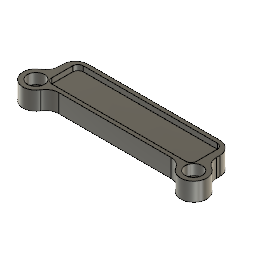
nametag (Autodesk Fusion 360 design; units mm, degrees)
Autodesk Fusion 360 part; units mm, degrees
note: some values were not read from the file. Set by a fixed rule: which sketch regions a step uses.
sketch "Sketch1" plane through (0, 0, 0) normal (0, 0, 1) x (1, 0, 0) in component "node_nametag"
  circle A0 centre (-64.8296, 1.0244) radius 1.75
  circle A1 centre (-4.8296, 1.0244) radius 1.75
  circle A2 centre (-64.8296, 1.0244) radius 5
  circle A3 centre (-4.8296, 1.0244) radius 5
  line L0 (-64.8296, 16.0244) -> (-4.8296, 16.0244)
  line L1 (-4.8296, 16.0244) -> (-4.8296, 1.0244)
  line L2 (-4.8296, 1.0244) -> (-64.8296, 1.0244)
  line L3 (-64.8296, 1.0244) -> (-64.8296, 16.0244)
  dimension "d1" = 3.5
  dimension "d2" = 3.5
  dimension "d3" = 60
  dimension "d4" = 10
  dimension "d5" = 10
  dimension "d6" = 15
  constraint horizontal A0.centre A1.centre
  constraint concentric A0 A2
  constraint concentric A1 A3
  constraint horizontal L0
  constraint vertical L1
  constraint horizontal L2
  constraint vertical L3
  constraint coincident A1.centre A3.centre
  constraint vertical A0.centre L0.start
  measures "d1" diameter of A0
  measures "d2" diameter of A1
  measures "d3" horizontal distance of A0.centre A1.centre
  measures "d4" diameter of A2
  measures "d5" diameter of A3
  measures "d6" distance of L0 L2
extrude "Extrude1" add sketch "Sketch1" along normal blind 5 contours A0 A2 L2 L3 | A0 A2 L2 L3 | A2 A3 L0 L1 L2 L3 | A1 A3 L1 L2 | A1 A3 L1 L2 in component "node_nametag"
sketch "Sketch2" plane through (0, 0, 5) normal (0, 0, 1) x (-1, 0, 0) in component "node_nametag"
  circle A0 centre (4.8296, -1.0244) radius 1.75
  circle A1 centre (64.8296, -1.0244) radius 1.75
  line L0 (64.8296, -16.0244) -> (64.8296, -6.0244)
  arc A2 (64.8296, -6.0244) -> (59.8296, -1.0244) centre (64.8296, -1.0244) ccw
  line L1 (59.8296, -1.0244) -> (9.8296, -1.0244)
  arc A3 (9.8296, -1.0244) -> (4.8296, -6.0244) centre (4.8296, -1.0244) ccw
  line L2 (4.8296, -6.0244) -> (4.8296, -16.0244)
  line L3 (4.8296, -16.0244) -> (64.8296, -16.0244)
  line L4 (62.3296, -14.5244) -> (7.3296, -14.5244)
  line L5 (7.3296, -14.5244) -> (7.3296, -2.5244)
  line L6 (7.3296, -2.5244) -> (62.3296, -2.5244)
  line L7 (62.3296, -2.5244) -> (62.3296, -14.5244)
  line L8 (34.8296, -16.0244) -> (34.8296, -1.0244) construction
  line L9 (64.8296, -11.0244) -> (4.8296, -11.0244) construction
  dimension "d9" = 12
  dimension "d10" = 55
  dimension "d11" = 27.5
  dimension "d12" = 1.5
  constraint horizontal L4
  constraint vertical L5
  constraint horizontal L6
  constraint vertical L7
  constraint midpoint L3 L8.start
  constraint midpoint L1 L8.end
  constraint midpoint L0 L9.start
  constraint midpoint L2 L9.end
  measures "d9" distance of L4 L6
  measures "d10" distance of L4.start L4.end
  measures "d11" distance of L7 L8
  measures "d12" distance of L3 L4
extrude "Extrude2" add sketch "Sketch2" along normal blind 2 in component "node_nametag"
fillet "Fillet1" radius 5 6 edges at (-4.8296, 16.0244, 3.5) (-64.8296, 16.0244, 3.5) (-59.8296, 1.0244, 3.5) (-9.8296, 1.0244, 3.5) (-64.8296, 6.0244, 3.5) (-4.8296, 6.0244, 3.5) in component "node_nametag"
fillet "Fillet1" radius 2 4 edges at (-62.3296, 14.5244, 6) (-62.3296, 2.5244, 6) (-7.3296, 2.5244, 6) (-7.3296, 14.5244, 6) in component "node_nametag"
sketch "Sketch3" plane through (0, 0, 7) normal (0, 0, 1) x (-1, 0, 0) in component "node_nametag"
  line L0 (9.3296, -2.5244) -> (60.3296, -2.5244)
  arc A0 (62.3296, -4.5244) -> (60.3296, -2.5244) centre (60.3296, -4.5244) ccw
  line L1 (62.3296, -4.5244) -> (62.3296, -12.5244)
  arc A1 (60.3296, -14.5244) -> (62.3296, -12.5244) centre (60.3296, -12.5244) ccw
  line L2 (60.3296, -14.5244) -> (9.3296, -14.5244)
  arc A2 (7.3296, -12.5244) -> (9.3296, -14.5244) centre (9.3296, -12.5244) ccw
  line L3 (7.3296, -12.5244) -> (7.3296, -4.5244)
  arc A3 (9.3296, -2.5244) -> (7.3296, -4.5244) centre (9.3296, -4.5244) ccw
  circle A4 centre (4.8296, -1.0244) radius 1.75
  circle A5 centre (64.8296, -1.0244) radius 1.75
  arc A6 (59.8296, -16.0244) -> (64.8296, -11.0244) centre (59.8296, -11.0244) ccw
  line L4 (64.8296, -11.0244) -> (64.8296, -9.6847)
  arc A7 (67.3296, -5.3546) -> (64.8296, -9.6847) centre (69.8296, -9.6847) ccw
  arc A8 (67.3296, -5.3546) -> (60.4995, 1.4756) centre (64.8296, -1.0244) ccw
  arc A9 (56.1694, -1.0244) -> (60.4995, 1.4756) centre (56.1694, 3.9756) ccw
  line L5 (56.1694, -1.0244) -> (13.4899, -1.0244)
  arc A10 (9.1597, 1.4756) -> (13.4899, -1.0244) centre (13.4899, 3.9756) ccw
  arc A11 (9.1597, 1.4756) -> (2.3296, -5.3546) centre (4.8296, -1.0244) ccw
  arc A12 (4.8296, -9.6847) -> (2.3296, -5.3546) centre (-0.1704, -9.6847) ccw
  line L6 (4.8296, -9.6847) -> (4.8296, -11.0244)
  arc A13 (4.8296, -11.0244) -> (9.8296, -16.0244) centre (9.8296, -11.0244) ccw
  line L7 (9.8296, -16.0244) -> (59.8296, -16.0244)
  circle A14 centre (4.8296, -1.0244) radius 3.25
  circle A15 centre (64.8296, -1.0244) radius 3.25
  dimension "d19" = 6.5
  dimension "d20" = 6.5
  constraint concentric A4 A14
  constraint concentric A5 A15
  measures "d19" diameter of A14
  measures "d20" diameter of A15
extrude "Extrude3" cut sketch "Sketch3" against normal blind 4 contours A14 | A15 in component "node_nametag"
component "node_nametag" placed x (1, 0, 0) y (0, 1, 0) z (0, 0, 1) at (0, 0, 0)
equation "d3 = ( 15 * 4 ) * 1 mm"
equation "d11 = d10 / 2"
